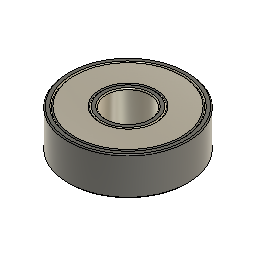
Eyes 130 (Autodesk Fusion 360 archive; units mm, degrees)
design "Roulement_8x22x7"
Autodesk Fusion 360 part; units mm, degrees
sketch "Sketch1" plane through (0, 0, 0) normal (0, 0, 1) x (1, 0, 0)
  circle A0 centre (0, 0) radius 11
  circle A1 centre (0, 0) radius 4
  circle A2 centre (0, 0) radius 10
  circle A3 centre (0, 0) radius 5
  dimension "d1" = 22
  dimension "d2" = 8
  dimension "d5" = -1
  dimension "d6" = 1
  constraint coincident A0.centre A1.centre
  measures "d1" diameter of A0
  measures "d2" diameter of A1
extrude "Extrude2" add sketch "Sketch1" along normal blind 7 contours A0 makes body 1
fillet "Fillet1" radius 0.2 2 edges at (-10.2556, -3.9778, 7) (-9.3233, 3.6162, 7) on bodies 1
fillet "Fillet1" radius 0.2 2 edges at (-10.2556, -3.9778, 0) (-9.3233, 3.6162, 0) on bodies 1
extrude "Extrude3" add sketch "Sketch1" along normal blind 7 separate body contours A3 makes body 2
fillet "Fillet2" radius 0.2 2 edges at (-4.6616, -1.8081, 7) (-3.7293, 1.4465, 7) on bodies 2
fillet "Fillet2" radius 0.2 2 edges at (-4.6616, -1.8081, 0) (-3.7293, 1.4465, 0) on bodies 2
extrude "Extrude4" add sketch "Sketch1" along normal blind 7 separate body contours A2 makes body 3
fillet "Fillet3" radius 0.2 2 edges at (-9.3233, -3.6162, 7) (-4.6616, 1.8081, 7) on bodies 3
fillet "Fillet3" radius 0.2 2 edges at (-9.3233, -3.6162, 0) (-4.6616, 1.8081, 0) on bodies 3
combine "Combine1" operation add target body 1 tool bodies 2 3
